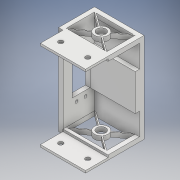
# Autodesk Inventor part: Biceps2 v2
Saved by Autodesk Inventor 2018 (Build 220112000, 112)
## iProperties
Created: 2018-04-10
Part Number: Biceps2 v2
Material: Plastique ABS
Document SubType Name: Modeling
Designer: Thomas
Density: 1.06 g/cm^3
Appearance: Lisse - Blanc
Author: Thomas
Autodesk Inventor part; units mm, degrees
ref_plane "YZ Plane" through (0, 0, 0) normal (1, 0, 0) x (0, 1, 0)
ref_plane "XZ Plane" through (0, 0, 0) normal (0, 1, 0) x (-1, 0, 0)
ref_plane "XY Plane" through (0, 0, 0) normal (0, 0, 1) x (1, 0, 0)
sketch "Esquisse1" plane through (0, 0, 0) normal (0, 0, 1) x (1, 0, 0)
  line L0 (0, 0) -> (50, 0)
  line L1 (50, 0) -> (50, -60)
  line L2 (50, -60) -> (0, -60)
  line L3 (0, -60) -> (0, 0)
  dimension "d0" = 50
  dimension "d1" = 60
  constraints: 8 end point, 2 parallel, 1 horizontal, 1 perpendicular
  measures "d0" distance of L1.end L2.end
  measures "d1" distance of L2.end L0.start
extrude "Extrusion1" add sketch "Esquisse1" along normal blind 5
sketch "Esquisse2" plane through (0, 0, 0) normal (0, 0, -1) x (-1, 0, 0)
  line L0 (0, -60) -> (-50, -60)
  line L1 (-50, -60) -> (-50, -35)
  line L2 (-50, -35) -> (0, -35)
  line L3 (0, -35) -> (0, -60)
  dimension "d4" = 25
  constraints: 8 end point, 2 parallel, 1 horizontal, 1 perpendicular
  measures "d4" distance of L0.end L1.end
extrude "Extrusion2" cut sketch "Esquisse2" against normal blind 2.5
sketch "Esquisse4" plane through (0, 0, 2.5) normal (0, 0, -1) x (-1, 0, 0)
  circle A0 centre (-10, -47.5) radius 2.6
  circle A1 centre (-40, -47.5) radius 2.6
  line L0 (-50, -60) -> (-50, -35) projected
  line L1 (0, -35) -> (0, -60) projected
  line L2 (0, -60) -> (-50, -60) projected
  point P0 (0, 0)
  dimension "d7" = 10
  dimension "d8" = 10
  dimension "d9" = 5.2
  dimension "d10" = 5.2
  dimension "d11" = 12.5
  dimension "d12" = 12.5
  constraints: 2 centre point
  measures "d7" distance from line of L0 A1.centre
  measures "d8" distance from line of L1 A0.centre
  measures "d9" diameter of A1
  measures "d10" diameter of A0
  measures "d11" distance from line of L2 A1.centre
  measures "d12" distance from line of L2 A0.centre
extrude "Extrusion3" cut sketch "Esquisse4" against normal blind 2.5
sketch "Esquisse5" plane through (0, 0, 0) normal (0, 1, 0) x (1, 0, 0)
  line L0 (0, -5) -> (50, -5)
  line L1 (50, -5) -> (50, 95)
  line L2 (50, 95) -> (0, 95)
  line L3 (0, 95) -> (0, -5)
  point P0 (0, 0)
  dimension "d15" = 50
  dimension "d16" = 100
  constraints: 8 end point, 2 parallel, 1 horizontal, 1 perpendicular
  measures "d15" distance of L0.start L0.end
  measures "d16" distance of L0.end L1.end
extrude "Extrusion4" add sketch "Esquisse5" along normal blind 5
sketch "Esquisse6" plane through (0, 0, 0) normal (0, -1, 0) x (1, 0, 0)
  line L0 (50, -95) -> (0, -95)
  line L1 (0, -95) -> (0, -90)
  line L2 (0, -90) -> (50, -90)
  line L3 (50, -90) -> (50, -95)
  dimension "d19" = 5
  constraints: 8 end point, 2 parallel, 1 horizontal, 1 perpendicular
  measures "d19" distance of L0.end L1.end
extrude "Extrusion5" add sketch "Esquisse6" along normal blind 60
sketch "Esquisse7" plane through (0, 0, -90) normal (0, 0, 1) x (1, 0, 0)
  line L0 (50, -60) -> (0, -60)
  line L1 (0, -60) -> (0, -35)
  line L2 (0, -35) -> (50, -35)
  line L3 (50, -35) -> (50, -60)
  point P0 (0, 0)
  dimension "d22" = 25
  constraints: 8 end point, 2 parallel, 1 horizontal, 1 perpendicular
  measures "d22" distance of L0.end L1.end
extrude "Extrusion6" cut sketch "Esquisse7" against normal blind 2.5
sketch "Esquisse8" plane through (0, 0, -92.5) normal (0, 0, 1) x (1, 0, 0)
  circle A0 centre (40, -47.5) radius 2.6
  circle A1 centre (10, -47.5) radius 2.6
  line L0 (50, -60) -> (0, -60) projected
  line L1 (0, -60) -> (0, -35) projected
  line L2 (50, -35) -> (50, -60) projected
  point P0 (0, 0)
  dimension "d25" = 5.2
  dimension "d26" = 5.2
  dimension "d27" = 12.5
  dimension "d28" = 12.5
  dimension "d29" = 10
  dimension "d30" = 10
  constraints: 2 centre point
  measures "d25" diameter of A1
  measures "d26" diameter of A0
  measures "d27" distance from line of L0 A1.centre
  measures "d28" distance from line of L0 A0.centre
  measures "d29" distance from line of L1 A1.centre
  measures "d30" distance from line of L2 A0.centre
extrude "Extrusion7" cut sketch "Esquisse8" against normal blind 2.5
sketch "Esquisse9" plane through (0, -60, 2.5) normal (-1, 0, 0) x (0, 0, 1)
  line L0 (2.5, 0) -> (2.5, 65) projected
  line L1 (2.5, 65) -> (-97.5, 65) projected
  line L2 (2.5, 25.0215) -> (-97.5, 25.0215)
  line L3 (-97.5, 25.0215) -> (-97.5, 65)
  line L4 (-97.5, 65) -> (2.5, 65)
  line L5 (2.5, 65) -> (2.5, 25.0215)
  point P0 (-2.5, 60)
  constraints: 8 end point, 2 parallel, 1 horizontal, 1 perpendicular, 1 point on line
extrude "Extrusion8" add sketch "Esquisse9" along normal blind 5
sketch "Esquisse10" plane through (-5, -60, 2.5) normal (-1, 0, 0) x (0, 0, 1)
  line L0 (-27.25, 35.0215) -> (-67.75, 35.0215)
  line L1 (-67.75, 35.0215) -> (-67.75, 55.0215)
  line L2 (-67.75, 55.0215) -> (-27.25, 55.0215)
  line L3 (-27.25, 55.0215) -> (-27.25, 35.0215)
  circle A0 centre (-21.45, 40.0215) radius 1.6
  circle A1 centre (-21.45, 50.0215) radius 1.6
  circle A2 centre (-73.55, 40.0215) radius 1.6
  circle A3 centre (-73.55, 50.0215) radius 1.6
  line L4 (2.5, 25.0215) -> (2.5, 65) projected
  line L5 (-97.5, 25.0215) -> (2.5, 25.0215) projected
  dimension "d35" = 20
  dimension "d36" = 40.5
  dimension "d37" = 3.2
  dimension "d38" = 3.2
  dimension "d39" = 3.2
  dimension "d40" = 3.2
  dimension "d41" = 10
  dimension "d42" = 5
  dimension "d43" = 5.8
  dimension "d44" = 5.8
  dimension "d45" = 5
  dimension "d46" = 5
  dimension "d47" = 5.8
  dimension "d48" = 5.8
  dimension "d49" = 29.75
  dimension "d50" = 10
  constraints: 8 end point, 4 centre point, 2 parallel, 1 horizontal, 1 perpendicular
  measures "d35" distance of L2.end L0.start
  measures "d36" distance of L1.end L2.end
  measures "d37" diameter of A3
  measures "d38" diameter of A2
  measures "d39" diameter of A0
  measures "d40" diameter of A1
  measures "d41" distance of A0.centre A1.centre
  measures "d42" distance from line of L2 A1.centre
  measures "d43" distance from line of L3 A0.centre
  measures "d44" distance from line of L3 A1.centre
  measures "d45" distance from line of L2 A3.centre
  measures "d46" distance from line of L0 A2.centre
  measures "d47" distance from line of L1 A3.centre
  measures "d48" distance from line of L1 A2.centre
  measures "d49" distance between parallel lines of L3 L4
  measures "d50" distance between parallel lines of L5 L0
extrude "Extrusion9" cut sketch "Esquisse10" against normal blind 5
sketch "Esquisse12" plane through (0, -60, 2.5) normal (1, 0, 0) x (0, 0, -1)
  line L0 (67.8734, 60) -> (27.3734, 60)
  line L1 (27.3734, 60) -> (27.3734, 55.2)
  line L2 (27.3734, 55.2) -> (67.8734, 55.2)
  line L3 (67.8734, 55.2) -> (67.8734, 60)
  point P0 (2.5, 60)
  dimension "d56" = 4.8
  dimension "d57" = 40.5
  constraints: 8 end point, 2 parallel, 1 horizontal, 1 perpendicular
  measures "d56" distance of L0.end L1.end
  measures "d57" distance of L1.end L2.end
extrude "Extrusion11" add sketch "Esquisse12" along normal blind 50
sketch "Esquisse13" plane through (50, -60, -95) normal (0, 0, -1) x (-1, 0, 0)
  line L0 (55, 65) -> (55, 25.0215) construction
  line L1 (0, 65) -> (55, 65) construction
  line L2 (55, 25.0215) -> (0, 65) construction
  line L3 (0, 60) -> (0, 25) construction
  line L4 (55, 65) -> (0, 25) construction
  circle A0 centre (27.5, 45) radius 5
  circle A1 centre (27.5, 45) radius 7.5
  line L5 (50.0269, 28.6364) -> (50, 60)
  line L6 (50, 60) -> (5, 60)
  line L7 (5, 60) -> (5, 28.6364)
  line L8 (50.0269, 28.6364) -> (5, 28.6364)
  line L9 (50.0269, 28.6364) -> (33.5718, 40.5973)
  line L10 (32.8572, 39.7511) -> (48.1482, 28.6364)
  line L11 (5, 28.6364) -> (21.4385, 40.5832)
  line L12 (22.1491, 39.7448) -> (6.875, 28.6364)
  line L13 (5, 60) -> (20.8518, 48.4714)
  line L14 (6.8787, 60) -> (21.4385, 49.4168)
  line L15 (0, 60) -> (50, 60) projected
  line L16 (50, 60) -> (34.1482, 48.4714)
  line L17 (50, 60) -> (48.125, 60)
  line L18 (48.125, 60) -> (33.5655, 49.4113)
  dimension "d61" = 15
  dimension "d60" = 10
  dimension "d62" = 5
  constraints: 30 end point, 11 point on line, 2 perpendicular, 1 centre point, 1 coincident, 1 midpoint, 10 other
  measures "d60" diameter of A0
  measures "d62" distance between parallel lines of L3 L7
extrude "Extrusion12" cut sketch "Esquisse13" against normal blind 5 contours A0 | A1 L16 L5 L9 | A1 L14 L6 L18 | L10 L8 L12 A1 | A1 L11 L7 L13
sketch "Esquisse15" plane through (0, 0, 5) normal (0, 0, 1) x (1, 0, 0)
  line L0 (49.9941, 5.0518) -> (50.0216, -34.9407) construction
  line L1 (-5.0098, 4.9946) -> (49.9941, 5.0518) construction
  line L2 (50.0216, -34.9407) -> (-5.0098, 4.9946) construction
  line L3 (-5, 1.3813) -> (-5, -34.9439) construction
  line L4 (49.9941, 5.0518) -> (-5, -34.9439) construction
  circle A0 centre (22.4971, -14.9461) radius 5
  circle A1 centre (22.4971, -14.9461) radius 7.5
  line L5 (45.0151, -31.3076) -> (44.995, 0)
  line L6 (44.995, 0) -> (0, 0)
  line L7 (0, 0) -> (0, -31.3076)
  line L8 (45.0151, -31.3076) -> (0, -31.3076)
  line L9 (45.0151, -31.3076) -> (28.5574, -19.3645)
  line L10 (27.8517, -20.1975) -> (43.1363, -31.3076)
  line L11 (0, -31.3076) -> (16.4355, -19.3628)
  line L12 (17.1458, -20.2009) -> (1.8741, -31.3076)
  line L13 (0, 0) -> (15.8473, -11.4775)
  line L14 (1.8729, 0) -> (16.4172, -10.5546)
  line L15 (44.995, 0) -> (29.1456, -11.4751)
  line L16 (0, -34.9785) -> (0, 0) projected
  line L17 (43.0479, 0) -> (28.5626, -10.5348)
  line L18 (44.995, 0) -> (43.0479, 0)
  line L19 (0, 0) -> (50, 0) projected
  dimension "d73" = 15
  dimension "d72" = 10
  dimension "d74" = 5
  dimension "d77" = 0
  constraints: 34 end point, 9 point on line, 1 centre point, 1 coincident, 1 midpoint, 1 parallel, 1 perpendicular, 1 vertical, 15 other
  measures "d72" diameter of A0
  measures "d74" distance between parallel lines of L3 L7
  measures "d77" distance between parallel lines of L16 L7
extrude "Extrusion13" cut sketch "Esquisse15" against normal blind 10 contours A0 | A1 L15 L5 L9 | A1 L14 L6 L17 | L10 L8 L12 A1 | A1 L11 L7 L13
